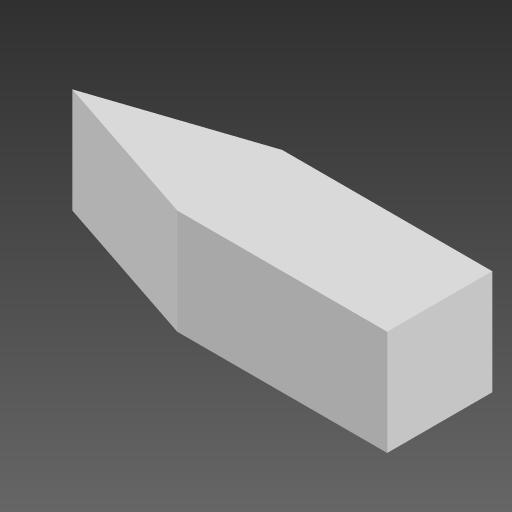
# Autodesk Inventor part: C3-2
Saved by Autodesk Inventor 2024 (Build 280153000, 153)
## iProperties
Created: 2024-06-03
Part Number: C3-2
Material: Generic
Document SubType Name: Modeling
Designer: brian
Density: 1 g/cm^3
Appearance: Default
Author: brian
Autodesk Inventor part; units mm, degrees
ref_plane "YZ Plane" through (0, 0, 0) normal (1, 0, 0) x (0, 1, 0)
ref_plane "XZ Plane" through (0, 0, 0) normal (0, 1, 0) x (-1, 0, 0)
ref_plane "XY Plane" through (0, 0, 0) normal (0, 0, 1) x (1, 0, 0)
sketch "Sketch1" plane through (0, 0, 0) normal (0, 1, 0) x (-1, 0, 0)
  line L0 (-609.6, -304.8) -> (609.6, -304.8)
  line L1 (609.6, -304.8) -> (609.6, 304.8) construction
  line L2 (609.6, 304.8) -> (-609.6, 304.8)
  line L3 (-609.6, 304.8) -> (-609.6, -304.8)
  line L4 (-609.6, -304.8) -> (609.6, 304.8) construction
  line L5 (609.6, -304.8) -> (-609.6, 304.8) construction
  line L6 (609.6, 304.8) -> (1524, 0)
  line L7 (1524, 0) -> (609.6, -304.8)
  line L8 (1524, 0) -> (609.6, 0) construction
  point P0 (0, 0)
  dimension "d0" = 1219.2
  dimension "d1" = 609.6
  dimension "d2" = 914.4
  constraints: 18 end point, 3 midpoint, 2 parallel, 1 equal length, 1 horizontal, 1 perpendicular
  measures "d0" distance of L0.start L0.end
  measures "d1" distance of L0.end L1.end
  measures "d2" distance from line of L1 L6.end
extrude "Extrusion1" add sketch "Sketch1" along normal blind 609.6
body "Solid1"
